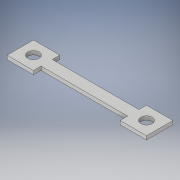
# Autodesk Inventor part: POE line bracket
Saved by Autodesk Inventor 2018 (Build 220112000, 112)
## iProperties
Created: 2019-11-08
Part Number: POE line bracket
Material: Generic
Document SubType Name: Modeling
Designer: Jacob
Density: 1 g/cm^3
Appearance: Default
Author: Jacob
Autodesk Inventor part; units mm, degrees
ref_plane "YZ Plane" through (0, 0, 0) normal (1, 0, 0) x (0, 1, 0)
ref_plane "XZ Plane" through (0, 0, 0) normal (0, 1, 0) x (-1, 0, 0)
ref_plane "XY Plane" through (0, 0, 0) normal (0, 0, 1) x (1, 0, 0)
sketch "Sketch1" plane through (0, 0, 0) normal (0, 1, 0) x (-1, 0, 0)
  line L0 (18.5, -1.5) -> (-18.5, -1.5)
  line L1 (-18.5, -1.5) -> (-18.5, 1.5)
  line L2 (-18.5, 1.5) -> (18.5, 1.5)
  line L3 (18.5, 1.5) -> (18.5, -1.5)
  line L4 (18.5, -1.5) -> (-18.5, 1.5) construction
  line L5 (-18.5, -1.5) -> (18.5, 1.5) construction
  point P0 (0, 0)
  dimension "d0" = 3
  dimension "d1" = 37
  constraints: 12 end point, 2 midpoint, 2 parallel, 1 horizontal, 1 perpendicular
  measures "d0" distance of L0.end L1.end
  measures "d1" distance of L0.start L0.end
extrude "Extrusion1" add sketch "Sketch1" along normal blind 1
sketch "Sketch2" plane through (0, 1, 0) normal (0, 1, 0) x (1, 0, 0)
  line L0 (-18.5, 1.5) -> (-18.5, -1.5) projected
  line L1 (-18.5, 0) -> (18.5, 0) construction
  line L2 (18.5, -1.5) -> (18.5, 1.5) projected
  line L3 (-18.5, 3.5) -> (-11.5, 3.5)
  line L4 (-11.5, 3.5) -> (-11.5, -3.5)
  line L5 (-11.5, -3.5) -> (-18.5, -3.5)
  line L6 (-18.5, -3.5) -> (-18.5, 3.5)
  line L7 (-18.5, 3.5) -> (-11.5, -3.5) construction
  line L8 (-11.5, 3.5) -> (-18.5, -3.5) construction
  line L9 (11.5, 3.5) -> (18.5, 3.5)
  line L10 (18.5, 3.5) -> (18.5, -3.5)
  line L11 (18.5, -3.5) -> (11.5, -3.5)
  line L12 (11.5, -3.5) -> (11.5, 3.5)
  line L13 (11.5, 3.5) -> (18.5, -3.5) construction
  line L14 (18.5, 3.5) -> (11.5, -3.5) construction
  point P0 (0, 0)
  point P1 (-15, 0)
  point P2 (15, 0)
  dimension "d4" = 7
  dimension "d5" = 7
  dimension "d6" = 0
  dimension "d7" = 7
  dimension "d8" = 7
  dimension "d9" = 0
  constraints: 26 end point, 6 midpoint, 4 parallel, 2 horizontal, 2 perpendicular, 2 point on line
  measures "d4" distance of L3.start L3.end
  measures "d5" distance of L3.end L4.end
  measures "d6" distance between parallel lines of L0 L6
  measures "d7" distance of L9.start L9.end
  measures "d8" distance of L11.end L9.start
  measures "d9" distance between parallel lines of L2 L10
extrude "Extrusion2" add sketch "Sketch2" against normal blind 1
sketch "Sketch3" plane through (0, 1, 0) normal (0, 1, 0) x (1, 0, 0)
  line L0 (-18.5, 3.5) -> (-11.5, 3.5) projected
  line L1 (-18.5, -3.5) -> (-18.5, 3.5) projected
  line L2 (-11.5, -3.5) -> (-18.5, -3.5) projected
  line L3 (-11.5, -1.5) -> (-11.5, -3.5) projected
  line L4 (-11.5, 3.5) -> (-11.5, 1.5) projected
  line L5 (11.5, 3.5) -> (18.5, 3.5) projected
  line L6 (18.5, 3.5) -> (18.5, -3.5) projected
  line L7 (18.5, -3.5) -> (11.5, -3.5) projected
  line L8 (11.5, -3.5) -> (11.5, -1.5) projected
  line L9 (11.5, 1.5) -> (11.5, 3.5) projected
  line L10 (11.5, 1.5) -> (-11.5, 1.5) projected
  line L11 (-11.5, 1.5) -> (-11.5, -1.5) construction
  line L12 (11.5, 1.5) -> (11.5, -1.5) construction
  line L13 (-11.5, 0) -> (-18.5, 0) construction
  line L14 (-18.5, 3.5) -> (-11.5, 3.5) projected
  line L15 (-15, 3.5) -> (-15, -3.5) construction
  line L16 (11.5, 0) -> (18.5, 0) construction
  line L17 (11.5, 3.5) -> (18.5, 3.5) projected
  line L18 (15, 3.5) -> (15, -3.5) construction
  line L19 (18.5, -3.5) -> (11.5, -3.5) projected
  circle A0 centre (-15, 0) radius 1.5
  circle A1 centre (15, 0) radius 1.5
  point P0 (0, 0)
  dimension "d14" = 3
  dimension "d15" = 3
  constraints: 12 end point, 10 midpoint, 2 centre point, 1 perpendicular, 1 vertical
  measures "d14" diameter of A0
  measures "d15" diameter of A1
extrude "Extrusion3" cut sketch "Sketch3" against normal blind 3
body "Solid1"
